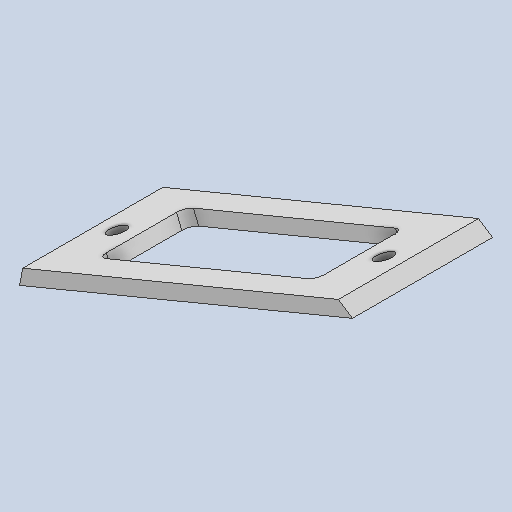
# Autodesk Inventor part: ДМФ 01 54 Нижний лист
Saved by Autodesk Inventor 2025 (Build 290162010, 162A)
## iProperties
Created: 2024-05-05
Part Number: ДМФ 01 54 Нижний лист
Material: Generic
Document SubType Name: Modeling
Designer: pokla
Density: 1 g/cm^3
Appearance: Default
Author: pokla
Autodesk Inventor part; units mm, degrees
ref_plane "YZ Plane" through (0, 0, 0) normal (1, 0, 0) x (0, 1, 0)
ref_plane "XZ Plane" through (0, 0, 0) normal (0, 1, 0) x (-1, 0, 0)
ref_plane "XY Plane" through (0, 0, 0) normal (0, 0, 1) x (1, 0, 0)
sketch "Sketch2" plane through (0, 0, 0) normal (0, 0, 1) x (1, 0, 0)
  line L0 (0, 277.6336) -> (196.3166, 196.3166) construction
  line L1 (196.3166, 196.3166) -> (277.6336, 0) construction
  line L2 (277.6336, 0) -> (196.3166, -196.3166) construction
  line L3 (196.3166, -196.3166) -> (0, -277.6336) construction
  line L4 (0, -277.6336) -> (-196.3166, -196.3166) construction
  line L5 (-196.3166, -196.3166) -> (-277.6336, 0) construction
  line L6 (-277.6336, 0) -> (-196.3166, 196.3166) construction
  line L7 (-196.3166, 196.3166) -> (0, 277.6336) construction
  line L8 (-196.3166, 196.3166) -> (0, 277.6336) construction
  line L9 (-461.2666, 773.8898) -> (-221.0579, 873.3874) construction
  line L10 (-98.1583, 236.9751) -> (-341.1623, 823.6386) construction
  line L11 (-221.0579, 873.3874) -> (0, 873.3874) construction
  line L12 (0, 873.3874) -> (0, 277.6336) construction
  line L13 (-461.2666, 773.8898) -> (-617.5782, 617.5782) construction
  line L14 (-617.5782, 617.5782) -> (-196.3166, 196.3166) construction
  line L15 (-5, 280.9745) -> (-195.1434, 202.2145) construction
  line L16 (-195.1434, 202.2145) -> (-610.5071, 617.5782) construction
  line L17 (-610.5071, 617.5782) -> (-458.4343, 769.651) construction
  line L18 (-458.4343, 769.651) -> (-220.0634, 868.3874) construction
  line L19 (-220.0634, 868.3874) -> (-5, 868.3874) construction
  line L20 (-5, 868.3874) -> (-5, 280.9745) construction
  line L21 (-13, 286.3199) -> (-193.2664, 211.6511) construction
  line L22 (-193.2664, 211.6511) -> (-599.1934, 617.5782) construction
  line L23 (-599.1934, 617.5782) -> (-453.9027, 762.8689) construction
  line L24 (-453.9027, 762.8689) -> (-218.4721, 860.3874) construction
  line L25 (-218.4721, 860.3874) -> (-13, 860.3874) construction
  line L26 (-13, 860.3874) -> (-13, 286.3199) construction
  line L27 (-5, 280.9745) -> (-195.1434, 202.2145)
  line L28 (-195.1434, 202.2145) -> (-193.2664, 211.6511)
  line L29 (-193.2664, 211.6511) -> (-13, 286.3199)
  line L30 (-13, 286.3199) -> (-5, 280.9745)
  point P0 (0, 0)
  point P1 (0, 0)
  point P2 (0, 0)
  dimension "d0" = 513
  dimension "d1" = 260
  dimension "d2" = 635
  dimension "d6" = 5
  dimension "d7" = 8
  constraints: 62 end point, 2 coincident, 2 midpoint, 2 parallel, 1 horizontal, 1 perpendicular, 1 symmetric about line, 1 vertical, 1 vertical alignment, 27 other
  measures "d0" distance between parallel lines of L5 L1
  measures "d1" distance of L9.start L11.start
  measures "d2" distance of L10.end L10.start
  measures "d6" distance between parallel lines of L12 L20
  measures "d7" distance between parallel lines of L20 L26
extrude "Extrusion1" add sketch "Sketch2" along normal mid plane 80
sketch "Sketch3" plane through (-13, 286.3199, -40) normal (-0.3827, 0.9239, 0) x (0.9239, 0.3827, 0)
  line L0 (-165.0595, -15) -> (-30.0595, -15)
  line L1 (-30.0595, -15) -> (-30.0595, -65)
  line L2 (-30.0595, -65) -> (-165.0595, -65)
  line L3 (-165.0595, -65) -> (-165.0595, -15)
  circle A0 centre (-15.0595, -40) radius 5
  circle A1 centre (-180.0595, -40) radius 5
  line L4 (0, -80) -> (-195.1189, -80) projected
  line L5 (-97.5595, -40) -> (-97.5595, -80) construction
  line L6 (5.3454, 0) -> (5.3454, -80) construction
  point P0 (-97.5595, -15)
  point P1 (-165.0595, -40)
  point P2 (-30.0595, -40)
  point P3 (5.3454, -40)
  dimension "d10" = 135
  dimension "d11" = 10
  dimension "d12" = 15
  dimension "d13" = 50
  constraints: 10 end point, 5 midpoint, 3 horizontal alignment, 2 centre point, 2 parallel, 2 perpendicular, 1 equal radius, 1 horizontal, 1 vertical alignment, 1 other
  measures "d10" distance of L0.start L0.end
  measures "d11" diameter of A1
  measures "d12" distance of point (-165.059, -40) A1.centre
  measures "d13" distance of L0.end L1.end
extrude "Extrusion2" cut sketch "Sketch3" against normal up to surface (8 mm away)
fillet "Fillet1" radius 5 4 edges at (-163.9643, 219.4589, -25) (-39.2406, 271.1211, -25) (-39.2406, 271.1211, 25) (-163.9643, 219.4589, 25)
equation "\"d0\" = Барабан_габарит_по_кассетам"
equation "\"d1\" = Кассета_длина_грани"
equation "\"d2\" = Кассета_высота"
equation "\"d10\" = Барабан_Длина_окна"
equation "\"d11\" = Кассета_Диам_шпильки"
equation "\"d13\" = Барабан_Ширина_окна"
equation "\"Барабан_габарит_по_кассетам\" = 513"
equation "\"Кассета_длина_грани\" = 260"
equation "\"Кассета_высота\" = 635"
equation "\"Барабан_Длина_окна\" = 135"
equation "\"Кассета_Диам_шпильки\" = 10"
equation "\"Барабан_Ширина_окна\" = 50"
body "Solid1"
